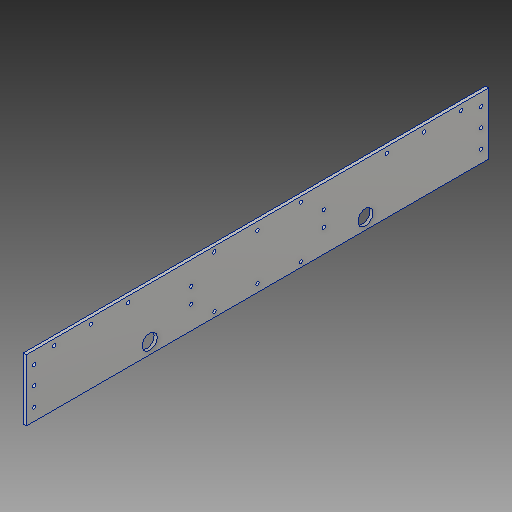
# Autodesk Inventor part: Bumper Plate
Saved by Autodesk Inventor 2019.4 (Build 234330000, 330)
## iProperties
Created: 2019-11-03
Part Number: Bumper Plate
Material: Aluminum 6061
Document SubType Name: Modeling
Designer: admin
Density: 2.7 g/cm^3
Appearance: Aluminum - Flat
Mass: 992.611 g
Surface Area: 1582.27 cm^2
Volume: 367.634 cm^3
Author: admin
Autodesk Inventor part; units mm, degrees
ref_plane "YZ Plane" through (0, 0, 0) normal (1, 0, 0) x (0, 1, 0)
ref_plane "XZ Plane" through (0, 0, 0) normal (0, 1, 0) x (-1, 0, 0)
ref_plane "XY Plane" through (0, 0, 0) normal (0, 0, 1) x (1, 0, 0)
sketch "Sketch1" plane through (0, 0, 0) normal (1, 0, 0) x (0, 1, 0)
  line L0 (-50, 375) -> (50, 375)
  line L1 (50, 375) -> (50, -375)
  line L2 (50, -375) -> (-50, -375)
  line L3 (-50, -375) -> (-50, 375)
  line L4 (-50, 375) -> (50, -375) construction
  line L5 (50, 375) -> (-50, -375) construction
  point P0 (0, 0)
  dimension "d0" = 100
  dimension "d1" = 750
  constraints: 12 end point, 2 midpoint, 2 parallel, 1 horizontal, 1 perpendicular
  measures "d0" distance of L1.end L2.end
  measures "d1" distance of L0.end L1.end
extrude "Extrusion1" add sketch "Sketch1" along normal blind 5
sketch "Sketch2" plane through (5, 0, 0) normal (1, 0, 0) x (0, 0, -1)
  circle A0 centre (-175, -31.7) radius 12.3
  line L0 (-375, -50) -> (375, -50) projected
  line L1 (-375, 50) -> (-375, -50) projected
  line L2 (375, 50) -> (-375, 50) projected
  line L3 (0, 50) -> (0, -50)
  circle A1 centre (175, -31.7) radius 12.3
  point P0 (0, 0)
  dimension "d4" = 18.3
  dimension "d5" = 200
  dimension "d6" = 24.6
  dimension "d9" = 375
  constraints: 2 centre point, 2 end point, 2 midpoint, 1 perpendicular, 1 symmetric about line, 1 other
  measures "d4" distance from line of L0 A0.centre
  measures "d5" distance from line of L1 A0.centre
  measures "d6" diameter of A0
  measures "d9" distance between parallel lines of L1 L3
extrude "Extrusion2" cut sketch "Sketch2" against normal through all contours A0 | A1
sketch "Sketch3" plane through (5, 0, 0) normal (1, 0, 0) x (0, 0, -1)
  circle A0 centre (70, -42) radius 2.75 projected
  circle A1 centre (0, -37.5) radius 2.75 projected
  circle A2 centre (70, 42) radius 2.75 projected
  circle A3 centre (0, 37.5) radius 2.75 projected
  circle A4 centre (330, 40.5) radius 2.75 projected
  circle A5 centre (-270, 40.5) radius 2.75 projected
  circle A6 centre (-210, 40.5) radius 2.75 projected
  circle A7 centre (362.5, 30) radius 2.75 projected
  circle A8 centre (-362.5, 30) radius 2.75 projected
  circle A9 centre (-362.5, 0) radius 2.75 projected
  circle A10 centre (107.5, 12.5) radius 2.75 projected
  circle A11 centre (-107.5, -12.5) radius 2.75 projected
  circle A12 centre (-107.5, 12.5) radius 2.75 projected
  circle A13 centre (107.5, -12.5) radius 2.75 projected
  circle A14 centre (-362.5, -30) radius 2.75 projected
  circle A15 centre (362.5, 0) radius 2.75 projected
  circle A16 centre (362.5, -30) radius 2.75 projected
  circle A17 centre (-330, 40.5) radius 2.75 projected
  circle A18 centre (210, 40.5) radius 2.75 projected
  circle A19 centre (270, 40.5) radius 2.75 projected
  circle A20 centre (-70, 42) radius 2.75 projected
  circle A21 centre (61.5777, -29.8129) radius 2.75 projected
  circle A22 centre (-70, -42) radius 2.75 projected
  circle A23 centre (-61.5777, -29.8129) radius 2.75 projected
  circle A24 centre (95.213, 6.296) radius 10.5 projected
  circle A25 centre (146.913, 6.296) radius 10.5 projected
  circle A26 centre (-95.213, 6.296) radius 10.5 projected
  circle A27 centre (-146.913, 6.296) radius 10.5 projected
  circle A28 centre (-55, -14) radius 10 projected
  circle A29 centre (-29.6, -14) radius 2.75 projected
  circle A30 centre (-80.4, -14) radius 2.75 projected
  circle A31 centre (-214.9997, -22.6996) radius 2.75 projected
  circle A32 centre (-97.163, -33.4172) radius 2.75 projected
  circle A33 centre (214.9997, -22.6996) radius 2.75 projected
  circle A34 centre (124.913, 42.776) radius 2.75 projected
  circle A35 centre (97.163, -33.4172) radius 2.75 projected
  circle A36 centre (80.4, -14) radius 2.75 projected
  circle A37 centre (29.6, -14) radius 2.75 projected
  circle A38 centre (55, 11.4) radius 2.75 projected
  circle A39 centre (55, -39.4) radius 2.75 projected
  circle A40 centre (61.5777, 29.8129) radius 2.75 projected
  circle A41 centre (186.913, 19.219) radius 2.75 projected
  circle A42 centre (-186.913, 19.219) radius 2.75 projected
  circle A43 centre (-124.913, 42.776) radius 2.75 projected
  circle A44 centre (-61.5777, 29.8129) radius 2.75 projected
  circle A45 centre (-55, 11.4) radius 2.75 projected
  circle A46 centre (-55, -39.4) radius 2.75 projected
  circle A47 centre (191, -31.7) radius 2.25 projected
  circle A48 centre (-191, -31.7) radius 2.25 projected
  circle A49 centre (-159, -31.7) radius 2.25 projected
  circle A50 centre (-175, -15.7) radius 2.25 projected
  circle A51 centre (175, -15.7) radius 2.25 projected
  circle A52 centre (159, -31.7) radius 2.25 projected
  circle A53 centre (-175, -31.7) radius 12.3 projected
  circle A54 centre (175, -31.7) radius 12.3 projected
  line L0 (-375, 50) -> (-375, -50) projected
  line L1 (-375, 50) -> (375, 50) projected
  line L2 (375, -50) -> (375, 50) projected
  line L3 (-375, -50) -> (375, -50) projected
  point P0 (0, 0)
extrude "Extrusion3" cut sketch "Sketch3" against normal blind 10 contours A0 | A1 | A2 | A3 | A4 | A5 | A6 | A7 | A8 | A9 | A10 | A11 | A12 | A13 | A14 | A15 | A16 | A17 | A18 | A19 | A20 | A22
body "Solid1"
